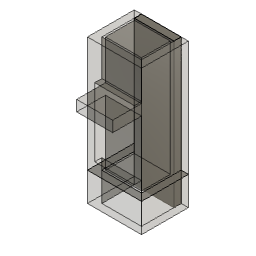
XOR Game v6 (Autodesk Fusion 360 archive; units mm, degrees)
design "Latch"
Autodesk Fusion 360 part; units mm, degrees
sketch "Sketch1" plane through (0, 0, 0) normal (0, 0, 1) x (1, 0, 0)
  line L0 (0, 0) -> (10, 0)
  line L1 (10, 0) -> (10, 8)
  line L2 (10, 8) -> (0, 8)
  line L3 (0, 8) -> (0, 0)
  line L4 (-0.5, 8.5) -> (10.5, 8.5)
  line L5 (10.5, 8.5) -> (10.5, -0.5)
  line L6 (10.5, -0.5) -> (-0.5, -0.5)
  line L7 (-0.5, -0.5) -> (-0.5, 8.5)
  line L8 (-2.5, 10.5) -> (12.5, 10.5)
  line L9 (12.5, 10.5) -> (12.5, -2.5)
  line L10 (12.5, -2.5) -> (-2.5, -2.5)
  line L11 (-2.5, -2.5) -> (-2.5, 10.5)
  dimension "d4" = 10
  dimension "d5" = 8
  dimension "d6" = 0.5
  dimension "d7" = 0.5
  dimension "d8" = 0.5
  dimension "d9" = 0.5
  dimension "d11" = 2
  dimension "d12" = 2
  dimension "d13" = 2
  dimension "d14" = 2
  constraint horizontal L0
  constraint vertical L1
  constraint horizontal L2
  constraint vertical L3
  constraint coincident L0.start L3.end
  constraint horizontal L4
  constraint vertical L5
  constraint horizontal L6
  constraint vertical L7
  constraint horizontal L8
  constraint vertical L9
  constraint horizontal L10
  constraint vertical L11
  measures "d4" distance of L0.start L0.end
  measures "d5" distance of L0.start L2.end
  measures "d6" distance of L2 L4
  measures "d7" distance of L0 L6
  measures "d8" distance of L3 L7
  measures "d9" distance of L1 L5
  measures "d11" distance of L4 L8
  measures "d12" distance of L6 L10
  measures "d13" distance of L7 L11
  measures "d14" distance of L5 L9
extrude "Extrude1" add sketch "Sketch1" along normal blind 8 contours L8 L9 L10 L11 makes body 1
extrude "Extrude2" add sketch "Sketch1" along normal blind 40 separate body contours L0 L1 L2 L3 makes body 2
sketch "Sketch2" plane through (0, 0, 8) normal (0, 0, 1) x (-1, 0, 0)
  line L0 (-10.5, 0.5) -> (0.5, 0.5)
  line L1 (0.5, 0.5) -> (0.5, -8.5)
  line L2 (0.5, -8.5) -> (-10.5, -8.5)
  line L3 (-10.5, -8.5) -> (-10.5, 0.5)
  line L4 (2.5, 2.5) -> (-12.5, 2.5)
  line L5 (-12.5, 2.5) -> (-12.5, -10.5)
  line L6 (-12.5, -10.5) -> (2.5, -10.5)
  line L7 (2.5, -10.5) -> (2.5, 2.5)
extrude "Extrude3" add sketch "Sketch2" along normal up to surface (32 mm away) separate body makes body 3
sketch "Sketch3" plane through (0, -2.5, 0) normal (0, -1, 0) x (1, 0, 0)
  line L0 (-2.5, 8) -> (12.5, 8)
  line L1 (12.5, 8) -> (12.5, 40)
  line L2 (12.5, 40) -> (-2.5, 40)
  line L3 (-2.5, 40) -> (-2.5, 8)
  line L4 (10.5, 8) -> (-0.5, 8)
  line L5 (-0.5, 8) -> (-0.5, 40)
  line L6 (-0.5, 40) -> (10.5, 40)
  line L7 (10.5, 40) -> (10.5, 8)
  line L8 (-0.5, 30) -> (10.5, 30)
  line L9 (10.5, 30) -> (10.5, 11)
  line L10 (10.5, 11) -> (-0.5, 11)
  line L11 (-0.5, 11) -> (-0.5, 30)
  dimension "d21" = 10
  dimension "d22" = 3
  constraint horizontal L8
  constraint vertical L9
  constraint horizontal L10
  constraint vertical L11
  constraint coincident L7 L9.end
  constraint coincident L5 L8.start
  measures "d21" distance of L2 L8
  measures "d22" distance of L4 L10
extrude "Extrude4" cut sketch "Sketch3" against normal up to surface (2 mm away) contours L5 L7 L8 L9 L10 L11 bodies 3
sketch "Sketch4" plane through (0, 0, 0) normal (0, -1, 0) x (1, 0, 0)
  line L0 (0, 0) -> (10, 0)
  line L1 (10, 0) -> (10, 40)
  line L2 (10, 40) -> (0, 40)
  line L3 (0, 40) -> (0, 0)
  line L4 (-0.5, 11) -> (-0.5, 30)
  line L5 (-0.5, 30) -> (10.5, 30)
  line L6 (10.5, 30) -> (10.5, 11)
  line L7 (10.5, 11) -> (-0.5, 11)
  line L8 (12.5, 40) -> (-2.5, 40)
  line L9 (-2.5, 40) -> (-2.5, 8)
  line L10 (-2.5, 8) -> (12.5, 8)
  line L11 (12.5, 8) -> (12.5, 40)
  line L12 (0, 29) -> (10, 29)
  line L13 (10, 29) -> (10, 26)
  line L14 (10, 26) -> (0, 26)
  line L15 (0, 26) -> (0, 29)
  dimension "d26" = 3
  dimension "d27" = 1
  constraint horizontal L12
  constraint vertical L13
  constraint horizontal L14
  constraint vertical L15
  constraint coincident L3 L12.start
  measures "d26" distance of L12.start L14.end
  measures "d27" distance of L5 L12
extrude "Extrude5" add sketch "Sketch4" along normal blind 8 contours L1 L3 L12 L13 L14 L15 bodies 2
extrude "Extrude6" cut sketch "Sketch1" along normal up to surface (8 mm away) contours L0 L1 L2 L3 bodies 2
copy_body "Body->Comp1" bodies 2 removing the originals makes body 4 in component "Component"
copy_body "Body->Comp2" bodies 3 removing the originals makes body 5 in component "Component'"
extrude "Extrude1'" cut 1 faces at (3.1667, 8.5, 18.6667) along direction (0, 1, 0) blind 2 on bodies 5 bodies 5 in component "Component'"
extrude "Extrude7" cut 1 faces at (3.1667, 8.5, 2.6667) along direction (0, 1, 0) blind 2 on bodies 1 bodies 1
sketch "Sketch5" plane through (0, 10.5, 0) normal (0, 1, 0) x (-1, 0, 0)
  line L0 (-10.5, 8) -> (-10.5, 40)
  line L1 (-10.5, 40) -> (-12.5, 40)
  line L2 (-12.5, 40) -> (-12.5, 8)
  line L3 (-12.5, 8) -> (-10.5, 8)
  line L4 (-10.5, 0) -> (0.5, 0)
  line L5 (0.5, 0) -> (0.5, 8)
  line L6 (0.5, 8) -> (-10.5, 8)
  line L7 (-10.5, 8) -> (-10.5, 0)
  line L8 (-10.5, 30) -> (0.5, 30)
  line L9 (0.5, 30) -> (0.5, 40)
  line L10 (0.5, 40) -> (-10.5, 40)
  line L11 (-10.5, 40) -> (-10.5, 30)
  line L12 (-10.5, 40) -> (0.5, 40)
  line L13 (0.5, 40) -> (0.5, 0)
  line L14 (0.5, 0) -> (-10.5, 0)
  line L15 (-10.5, 0) -> (-10.5, 40)
  constraint horizontal L12
  constraint vertical L13
  constraint horizontal L14
  constraint vertical L15
  constraint coincident L4.end L5.start
  constraint coincident L0.end L1.start
extrude "Extrude8" add sketch "Sketch5" against normal blind 2 separate body contours L0 L6 L8 L13 L15 | L4 L5 L6 L7 L13 L14 L15 | L0 L8 L9 L10 L11 L12 L13 L15 makes body 6
component "Component" placed x (1, 0, 0) y (0, 1, 0) z (0, 0, 1) at (0, 0, 0)
component "Component'" placed x (1, 0, 0) y (0, 1, 0) z (0, 0, 1) at (0, 0, 0)
equation "Latch_width = 10 mm"
equation "Latch_height = 8 mm"
equation "Latch_gap = 0.5 mm"
equation "d4 = Latch_width"
equation "d5 = Latch_height"
equation "d6 = Latch_gap"
equation "d7 = Latch_gap"
equation "d8 = Latch_gap"
equation "d9 = Latch_gap"
equation "Latch_shell_thickness = 2 mm"
equation "d11 = Latch_shell_thickness"
equation "d12 = Latch_shell_thickness"
equation "d13 = Latch_shell_thickness"
equation "d14 = Latch_shell_thickness"
